Autodesk Fusion 360 part; units mm, degrees
(part 3 of 10)
sketch "草图3 (7)" plane through (727, 0, 0) normal (1, 0, 0) x (0, 0, -1) in component "R2_Integrated"
  line L0 (-20, 137) -> (-20, 165)
  line L1 (-20, 165) -> (-23, 165)
  line L2 (-23, 165) -> (-24.958, 137)
  line L3 (-24.958, 137) -> (-20, 137)
  dimension "d1011" = 23
  dimension "d1012" = 24.958
  constraint vertical L0
  constraint horizontal L1
  constraint horizontal L3
  measures "d1011" horizontal distance of origin L1.end
  measures "d1012" horizontal distance of origin L2.end
extrude "Drain tongue floor'''" add sketch "草图3 (7)" along normal blind 34 bodies 19 in component "R2_Integrated"
ref_plane "工作平面4" through (727, 0, 0) normal (1, 0, 0) x (0, 1, 0) in component "R2_Integrated"
sketch "草图4 (7)" plane through (727, 0, 0) normal (1, 0, 0) x (0, 0, -1) in component "R2_Integrated"
  line L0 (-20, 137) -> (-20, 165)
  line L1 (-20, 165) -> (-29, 165)
  line L2 (-29, 165) -> (-30.958, 137)
  line L3 (-30.958, 137) -> (-20, 137)
  dimension "d1020" = 29
  dimension "d1021" = 30.958
  constraint vertical L0
  constraint horizontal L1
  constraint horizontal L3
  measures "d1020" horizontal distance of origin L1.end
  measures "d1021" horizontal distance of origin L2.end
extrude "Tongue side rail'''" add sketch "草图4 (7)" along normal blind 3 bodies 19 in component "R2_Integrated"
ref_plane "工作平面5" through (758, 0, 0) normal (1, 0, 0) x (0, 1, 0) in component "R2_Integrated"
sketch "草图5 (7)" plane through (758, 0, 0) normal (1, 0, 0) x (0, 0, -1) in component "R2_Integrated"
  line L0 (-20, 137) -> (-20, 165)
  line L1 (-20, 165) -> (-29, 165)
  line L2 (-29, 165) -> (-30.958, 137)
  line L3 (-30.958, 137) -> (-20, 137)
  dimension "d1029" = 29
  dimension "d1030" = 30.958
  constraint vertical L0
  constraint horizontal L1
  constraint horizontal L3
  measures "d1029" horizontal distance of origin L1.end
  measures "d1030" horizontal distance of origin L2.end
extrude "Tongue side rail (1)'''" add sketch "草图5 (7)" along normal blind 3 bodies 19 in component "R2_Integrated"
ref_plane "工作平面6" through (730, 0, 0) normal (1, 0, 0) x (0, 1, 0) in component "R2_Integrated"
sketch "草图6 (7)" plane through (730, 0, 0) normal (1, 0, 0) x (0, 0, -1) in component "R2_Integrated"
  line L0 (-24.958, 137) -> (-23, 165)
  line L1 (-23, 165) -> (-41, 165)
  line L2 (-41, 165) -> (-41, 137)
  line L3 (-41, 137) -> (-24.958, 137)
  dimension "d1035" = 24.958
  dimension "d1037" = 23
  dimension "d1039" = 41
  constraint horizontal L1
  constraint vertical L2
  constraint horizontal L3
  measures "d1035" horizontal distance of origin L0.start
  measures "d1037" horizontal distance of origin L0.end
  measures "d1039" horizontal distance of origin L1.end
extrude "Open drain mouth'''" cut sketch "草图6 (7)" along normal blind 28 bodies 19 in component "R2_Integrated"
ref_plane "工作平面7" through (0, 0, 20) normal (0, 0, 1) x (1, 0, 0) in component "R2_Integrated"
sketch "草图7 (7)" plane through (0, 0, 20) normal (0, 0, 1) x (1, 0, 0) in component "R2_Integrated"
  line L0 (729, 53) -> (741, 53)
  line L1 (741, 53) -> (741, 65)
  line L2 (741, 65) -> (729, 65)
  line L3 (729, 65) -> (729, 53)
  dimension "d1044" = 729
  dimension "d1046" = 12
  dimension "d1047" = 12
  constraint horizontal L0
  constraint vertical L1
  constraint horizontal L2
  constraint vertical L3
  measures "d1044" horizontal distance of origin L0.start
  measures "d1046" horizontal distance of L0.start L0.end
  measures "d1047" vertical distance of L0.end L1.end
extrude "Grate seat 00'''" add sketch "草图7 (7)" along normal blind 16 bodies 19 in component "R2_Integrated"
ref_plane "工作平面8" through (0, 0, 20) normal (0, 0, 1) x (1, 0, 0) in component "R2_Integrated"
sketch "草图8 (7)" plane through (0, 0, 20) normal (0, 0, 1) x (1, 0, 0) in component "R2_Integrated"
  line L0 (761, 125) -> (773, 125)
  line L1 (773, 125) -> (773, 137)
  line L2 (773, 137) -> (761, 137)
  line L3 (761, 137) -> (761, 125)
  dimension "d1052" = 761
  dimension "d1053" = 125
  dimension "d1054" = 12
  dimension "d1055" = 12
  constraint horizontal L0
  constraint vertical L1
  constraint horizontal L2
  constraint vertical L3
  measures "d1052" horizontal distance of origin L0.start
  measures "d1053" vertical distance of origin L0.start
  measures "d1054" horizontal distance of L0.start L0.end
  measures "d1055" vertical distance of L0.end L1.end
extrude "Grate seat 01'''" add sketch "草图8 (7)" along normal blind 16 bodies 19 in component "R2_Integrated"
ref_plane "工作平面9" through (0, 0, 20) normal (0, 0, 1) x (1, 0, 0) in component "R2_Integrated"
sketch "草图9 (7)" plane through (0, 0, 20) normal (0, 0, 1) x (1, 0, 0) in component "R2_Integrated"
  line L0 (845, 53) -> (857, 53)
  line L1 (857, 53) -> (857, 65)
  line L2 (857, 65) -> (845, 65)
  line L3 (845, 65) -> (845, 53)
  dimension "d1060" = 845
  dimension "d1062" = 12
  dimension "d1063" = 12
  constraint horizontal L0
  constraint vertical L1
  constraint horizontal L2
  constraint vertical L3
  measures "d1060" horizontal distance of origin L0.start
  measures "d1062" horizontal distance of L0.start L0.end
  measures "d1063" vertical distance of L0.end L1.end
extrude "Grate seat 10'''" add sketch "草图9 (7)" along normal blind 16 bodies 19 in component "R2_Integrated"
ref_plane "工作平面10" through (0, 0, 20) normal (0, 0, 1) x (1, 0, 0) in component "R2_Integrated"
sketch "草图10 (7)" plane through (0, 0, 20) normal (0, 0, 1) x (1, 0, 0) in component "R2_Integrated"
  line L0 (845, 125) -> (857, 125)
  line L1 (857, 125) -> (857, 137)
  line L2 (857, 137) -> (845, 137)
  line L3 (845, 137) -> (845, 125)
  dimension "d1068" = 845
  dimension "d1069" = 125
  dimension "d1070" = 12
  dimension "d1071" = 12
  constraint horizontal L0
  constraint vertical L1
  constraint horizontal L2
  constraint vertical L3
  measures "d1068" horizontal distance of origin L0.start
  measures "d1069" vertical distance of origin L0.start
  measures "d1070" horizontal distance of L0.start L0.end
  measures "d1071" vertical distance of L0.end L1.end
extrude "Grate seat 11'''" add sketch "草图10 (7)" along normal blind 16 bodies 19 in component "R2_Integrated"
ref_plane "工作平面11" through (727, 0, 0) normal (1, 0, 0) x (0, 1, 0) in component "R2_Integrated"
sketch "草图11 (7)" plane through (727, 0, 0) normal (1, 0, 0) x (0, 0, -1) in component "R2_Integrated"
  line L0 (-19.8, 163) -> (-19.8, 164)
  line L1 (-19.8, 164) -> (-20.6, 164)
  line L2 (-20.6, 164) -> (-20.6, 163)
  line L3 (-20.6, 163) -> (-19.8, 163)
  dimension "d1076" = 19.8
  dimension "d1077" = 163
  dimension "d1078" = 164
  dimension "d1079" = 20.6
  constraint vertical L0
  constraint horizontal L1
  constraint vertical L2
  constraint horizontal L3
  measures "d1076" horizontal distance of origin L0.start
  measures "d1077" vertical distance of origin L0.start
  measures "d1078" vertical distance of origin L0.end
  measures "d1079" horizontal distance of origin L1.end
extrude "Drip break underside groove'''" cut sketch "草图11 (7)" along normal blind 34 bodies 19 in component "R2_Integrated"
ref_plane "工作平面12" through (0, 0, 20) normal (0, 0, 1) x (1, 0, 0) in component "R2_Integrated"
sketch "草图12 (7)" plane through (0, 0, 20) normal (0, 0, 1) x (1, 0, 0) in component "R2_Integrated"
  line L0 (732.75, 56.75) -> (741.25, 56.75)
  line L1 (741.25, 56.75) -> (741.25, 65.25)
  line L2 (741.25, 65.25) -> (732.75, 65.25)
  line L3 (732.75, 65.25) -> (732.75, 56.75)
  dimension "d1084" = 732.75
  dimension "d1085" = 56.75
  dimension "d1086" = 8.5
  dimension "d1087" = 8.5
  constraint horizontal L0
  constraint vertical L1
  constraint horizontal L2
  constraint vertical L3
  measures "d1084" horizontal distance of origin L0.start
  measures "d1085" vertical distance of origin L0.start
  measures "d1086" horizontal distance of L0.start L0.end
  measures "d1087" vertical distance of L0.end L1.end
extrude "Foot socket 00'''" cut sketch "草图12 (7)" along normal blind 1.8 bodies 19 in component "R2_Integrated"
ref_plane "工作平面13" through (0, 0, 20) normal (0, 0, 1) x (1, 0, 0) in component "R2_Integrated"
sketch "草图13 (7)" plane through (0, 0, 20) normal (0, 0, 1) x (1, 0, 0) in component "R2_Integrated"
  line L0 (732.75, 118.75) -> (741.25, 118.75)
  line L1 (741.25, 118.75) -> (741.25, 127.25)
  line L2 (741.25, 127.25) -> (732.75, 127.25)
  line L3 (732.75, 127.25) -> (732.75, 118.75)
  dimension "d1092" = 732.75
  dimension "d1093" = 118.75
  dimension "d1094" = 8.5
  dimension "d1095" = 8.5
  constraint horizontal L0
  constraint vertical L1
  constraint horizontal L2
  constraint vertical L3
  measures "d1092" horizontal distance of origin L0.start
  measures "d1093" vertical distance of origin L0.start
  measures "d1094" horizontal distance of L0.start L0.end
  measures "d1095" vertical distance of L0.end L1.end
extrude "Foot socket 01'''" cut sketch "草图13 (7)" along normal blind 1.8 bodies 19 in component "R2_Integrated"
ref_plane "工作平面14" through (0, 0, 20) normal (0, 0, 1) x (1, 0, 0) in component "R2_Integrated"
sketch "草图14 (6)" plane through (0, 0, 20) normal (0, 0, 1) x (1, 0, 0) in component "R2_Integrated"
  line L0 (844.75, 56.75) -> (853.25, 56.75)
  line L1 (853.25, 56.75) -> (853.25, 65.25)
  line L2 (853.25, 65.25) -> (844.75, 65.25)
  line L3 (844.75, 65.25) -> (844.75, 56.75)
  dimension "d1100" = 844.75
  dimension "d1101" = 56.75
  dimension "d1102" = 8.5
  dimension "d1103" = 8.5
  constraint horizontal L0
  constraint vertical L1
  constraint horizontal L2
  constraint vertical L3
  measures "d1100" horizontal distance of origin L0.start
  measures "d1101" vertical distance of origin L0.start
  measures "d1102" horizontal distance of L0.start L0.end
  measures "d1103" vertical distance of L0.end L1.end
extrude "Foot socket 10'''" cut sketch "草图14 (6)" along normal blind 1.8 bodies 19 in component "R2_Integrated"
ref_plane "工作平面15" through (0, 0, 20) normal (0, 0, 1) x (1, 0, 0) in component "R2_Integrated"
sketch "草图15 (6)" plane through (0, 0, 20) normal (0, 0, 1) x (1, 0, 0) in component "R2_Integrated"
  line L0 (844.75, 118.75) -> (853.25, 118.75)
  line L1 (853.25, 118.75) -> (853.25, 127.25)
  line L2 (853.25, 127.25) -> (844.75, 127.25)
  line L3 (844.75, 127.25) -> (844.75, 118.75)
  dimension "d1108" = 844.75
  dimension "d1109" = 118.75
  dimension "d1110" = 8.5
  dimension "d1111" = 8.5
  constraint horizontal L0
  constraint vertical L1
  constraint horizontal L2
  constraint vertical L3
  measures "d1108" horizontal distance of origin L0.start
  measures "d1109" vertical distance of origin L0.start
  measures "d1110" horizontal distance of L0.start L0.end
  measures "d1111" vertical distance of L0.end L1.end
extrude "Foot socket 11'''" cut sketch "草图15 (6)" along normal blind 1.8 bodies 19 in component "R2_Integrated"
ref_plane "工作平面1" through (0, 0, 36) normal (0, 0, 1) x (1, 0, 0) in component "R2_RemovableGrate"
sketch "草图1 (20)" plane through (0, 0, 36) normal (0, 0, 1) x (1, 0, 0) in component "R2_RemovableGrate"
  line L0 (729.3, 53.3) -> (856.7, 53.3)
  line L1 (856.7, 53.3) -> (856.7, 136.7)
  line L2 (856.7, 136.7) -> (729.3, 136.7)
  line L3 (729.3, 136.7) -> (729.3, 53.3)
  dimension "d1116" = 729.3
  dimension "d1118" = 127.4
  dimension "d1119" = 83.4
  constraint horizontal L0
  constraint vertical L1
  constraint horizontal L2
  constraint vertical L3
  measures "d1116" horizontal distance of origin L0.start
  measures "d1118" horizontal distance of L0.start L0.end
  measures "d1119" vertical distance of L0.end L1.end
extrude "Horizontal removable deck'''" add sketch "草图1 (20)" along normal blind 4 separate body makes body 20 in component "R2_RemovableGrate"
ref_plane "工作平面2" through (0, 0, 36) normal (0, 0, 1) x (1, 0, 0) in component "R2_RemovableGrate"
sketch "草图2 (20)" plane through (0, 0, 36) normal (0, 0, 1) x (1, 0, 0) in component "R2_RemovableGrate"
  line L0 (741, 60.3) -> (745, 60.3)
  line L1 (745, 60.3) -> (745, 129.7)
  line L2 (745, 129.7) -> (741, 129.7)
  line L3 (741, 129.7) -> (741, 60.3)
  dimension "d1124" = 741
  dimension "d1126" = 4
  dimension "d1127" = 69.4
  constraint horizontal L0
  constraint vertical L1
  constraint horizontal L2
  constraint vertical L3
  measures "d1124" horizontal distance of origin L0.start
  measures "d1126" horizontal distance of L0.start L0.end
  measures "d1127" vertical distance of L0.end L1.end
extrude "Drain slot 1'''" cut sketch "草图2 (20)" along normal blind 4 bodies 20 in component "R2_RemovableGrate"
ref_plane "工作平面3" through (0, 0, 36) normal (0, 0, 1) x (1, 0, 0) in component "R2_RemovableGrate"
sketch "草图3 (8)" plane through (0, 0, 36) normal (0, 0, 1) x (1, 0, 0) in component "R2_RemovableGrate"
  line L0 (751, 60.3) -> (755, 60.3)
  line L1 (755, 60.3) -> (755, 129.7)
  line L2 (755, 129.7) -> (751, 129.7)
  line L3 (751, 129.7) -> (751, 60.3)
  dimension "d1132" = 751
  dimension "d1134" = 4
  dimension "d1135" = 69.4
  constraint horizontal L0
  constraint vertical L1
  constraint horizontal L2
  constraint vertical L3
  measures "d1132" horizontal distance of origin L0.start
  measures "d1134" horizontal distance of L0.start L0.end
  measures "d1135" vertical distance of L0.end L1.end
extrude "Drain slot 2'''" cut sketch "草图3 (8)" along normal blind 4 bodies 20 in component "R2_RemovableGrate"
ref_plane "工作平面4" through (0, 0, 36) normal (0, 0, 1) x (1, 0, 0) in component "R2_RemovableGrate"
sketch "草图4 (8)" plane through (0, 0, 36) normal (0, 0, 1) x (1, 0, 0) in component "R2_RemovableGrate"
  line L0 (761, 60.3) -> (765, 60.3)
  line L1 (765, 60.3) -> (765, 129.7)
  line L2 (765, 129.7) -> (761, 129.7)
  line L3 (761, 129.7) -> (761, 60.3)
  dimension "d1140" = 761
  dimension "d1142" = 4
  dimension "d1143" = 69.4
  constraint horizontal L0
  constraint vertical L1
  constraint horizontal L2
  constraint vertical L3
  measures "d1140" horizontal distance of origin L0.start
  measures "d1142" horizontal distance of L0.start L0.end
  measures "d1143" vertical distance of L0.end L1.end
extrude "Drain slot 3'''" cut sketch "草图4 (8)" along normal blind 4 bodies 20 in component "R2_RemovableGrate"
ref_plane "工作平面5" through (0, 0, 36) normal (0, 0, 1) x (1, 0, 0) in component "R2_RemovableGrate"
sketch "草图5 (8)" plane through (0, 0, 36) normal (0, 0, 1) x (1, 0, 0) in component "R2_RemovableGrate"
  line L0 (771, 60.3) -> (775, 60.3)
  line L1 (775, 60.3) -> (775, 129.7)
  line L2 (775, 129.7) -> (771, 129.7)
  line L3 (771, 129.7) -> (771, 60.3)
  dimension "d1148" = 771
  dimension "d1150" = 4
  dimension "d1151" = 69.4
  constraint horizontal L0
  constraint vertical L1
  constraint horizontal L2
  constraint vertical L3
  measures "d1148" horizontal distance of origin L0.start
  measures "d1150" horizontal distance of L0.start L0.end
  measures "d1151" vertical distance of L0.end L1.end
extrude "Drain slot 4'''" cut sketch "草图5 (8)" along normal blind 4 bodies 20 in component "R2_RemovableGrate"
ref_plane "工作平面6" through (0, 0, 36) normal (0, 0, 1) x (1, 0, 0) in component "R2_RemovableGrate"
sketch "草图6 (8)" plane through (0, 0, 36) normal (0, 0, 1) x (1, 0, 0) in component "R2_RemovableGrate"
  line L0 (781, 60.3) -> (785, 60.3)
  line L1 (785, 60.3) -> (785, 129.7)
  line L2 (785, 129.7) -> (781, 129.7)
  line L3 (781, 129.7) -> (781, 60.3)
  dimension "d1156" = 781
  dimension "d1158" = 4
  dimension "d1159" = 69.4
  constraint horizontal L0
  constraint vertical L1
  constraint horizontal L2
  constraint vertical L3
  measures "d1156" horizontal distance of origin L0.start
  measures "d1158" horizontal distance of L0.start L0.end
  measures "d1159" vertical distance of L0.end L1.end
extrude "Drain slot 5'''" cut sketch "草图6 (8)" along normal blind 4 bodies 20 in component "R2_RemovableGrate"
ref_plane "工作平面7" through (0, 0, 36) normal (0, 0, 1) x (1, 0, 0) in component "R2_RemovableGrate"
sketch "草图7 (8)" plane through (0, 0, 36) normal (0, 0, 1) x (1, 0, 0) in component "R2_RemovableGrate"
  line L0 (791, 60.3) -> (795, 60.3)
  line L1 (795, 60.3) -> (795, 129.7)
  line L2 (795, 129.7) -> (791, 129.7)
  line L3 (791, 129.7) -> (791, 60.3)
  dimension "d1164" = 791
  dimension "d1166" = 4
  dimension "d1167" = 69.4
  constraint horizontal L0
  constraint vertical L1
  constraint horizontal L2
  constraint vertical L3
  measures "d1164" horizontal distance of origin L0.start
  measures "d1166" horizontal distance of L0.start L0.end
  measures "d1167" vertical distance of L0.end L1.end
extrude "Drain slot 6'''" cut sketch "草图7 (8)" along normal blind 4 bodies 20 in component "R2_RemovableGrate"
ref_plane "工作平面8" through (0, 0, 36) normal (0, 0, 1) x (1, 0, 0) in component "R2_RemovableGrate"
sketch "草图8 (8)" plane through (0, 0, 36) normal (0, 0, 1) x (1, 0, 0) in component "R2_RemovableGrate"
  line L0 (801, 60.3) -> (805, 60.3)
  line L1 (805, 60.3) -> (805, 129.7)
  line L2 (805, 129.7) -> (801, 129.7)
  line L3 (801, 129.7) -> (801, 60.3)
  dimension "d1172" = 801
  dimension "d1174" = 4
  dimension "d1175" = 69.4
  constraint horizontal L0
  constraint vertical L1
  constraint horizontal L2
  constraint vertical L3
  measures "d1172" horizontal distance of origin L0.start
  measures "d1174" horizontal distance of L0.start L0.end
  measures "d1175" vertical distance of L0.end L1.end
extrude "Drain slot 7'''" cut sketch "草图8 (8)" along normal blind 4 bodies 20 in component "R2_RemovableGrate"
ref_plane "工作平面9" through (0, 0, 36) normal (0, 0, 1) x (1, 0, 0) in component "R2_RemovableGrate"
sketch "草图9 (8)" plane through (0, 0, 36) normal (0, 0, 1) x (1, 0, 0) in component "R2_RemovableGrate"
  line L0 (811, 60.3) -> (815, 60.3)
  line L1 (815, 60.3) -> (815, 129.7)
  line L2 (815, 129.7) -> (811, 129.7)
  line L3 (811, 129.7) -> (811, 60.3)
  dimension "d1180" = 811
  dimension "d1182" = 4
  dimension "d1183" = 69.4
  constraint horizontal L0
  constraint vertical L1
  constraint horizontal L2
  constraint vertical L3
  measures "d1180" horizontal distance of origin L0.start
  measures "d1182" horizontal distance of L0.start L0.end
  measures "d1183" vertical distance of L0.end L1.end
extrude "Drain slot 8'''" cut sketch "草图9 (8)" along normal blind 4 bodies 20 in component "R2_RemovableGrate"
ref_plane "工作平面10" through (0, 0, 36) normal (0, 0, 1) x (1, 0, 0) in component "R2_RemovableGrate"
sketch "草图10 (8)" plane through (0, 0, 36) normal (0, 0, 1) x (1, 0, 0) in component "R2_RemovableGrate"
  line L0 (821, 60.3) -> (825, 60.3)
  line L1 (825, 60.3) -> (825, 129.7)
  line L2 (825, 129.7) -> (821, 129.7)
  line L3 (821, 129.7) -> (821, 60.3)
  dimension "d1188" = 821
  dimension "d1190" = 4
  dimension "d1191" = 69.4
  constraint horizontal L0
  constraint vertical L1
  constraint horizontal L2
  constraint vertical L3
  measures "d1188" horizontal distance of origin L0.start
  measures "d1190" horizontal distance of L0.start L0.end
  measures "d1191" vertical distance of L0.end L1.end
extrude "Drain slot 9'''" cut sketch "草图10 (8)" along normal blind 4 bodies 20 in component "R2_RemovableGrate"
ref_plane "工作平面11" through (0, 0, 36) normal (0, 0, 1) x (1, 0, 0) in component "R2_RemovableGrate"
sketch "草图11 (8)" plane through (0, 0, 36) normal (0, 0, 1) x (1, 0, 0) in component "R2_RemovableGrate"
  line L0 (831, 60.3) -> (835, 60.3)
  line L1 (835, 60.3) -> (835, 129.7)
  line L2 (835, 129.7) -> (831, 129.7)
  line L3 (831, 129.7) -> (831, 60.3)
  dimension "d1196" = 831
  dimension "d1198" = 4
  dimension "d1199" = 69.4
  constraint horizontal L0
  constraint vertical L1
  constraint horizontal L2
  constraint vertical L3
  measures "d1196" horizontal distance of origin L0.start
  measures "d1198" horizontal distance of L0.start L0.end
  measures "d1199" vertical distance of L0.end L1.end
extrude "Drain slot 10'''" cut sketch "草图11 (8)" along normal blind 4 bodies 20 in component "R2_RemovableGrate"
ref_plane "工作平面12" through (0, 0, 36) normal (0, 0, 1) x (1, 0, 0) in component "R2_RemovableGrate"
sketch "草图12 (8)" plane through (0, 0, 36) normal (0, 0, 1) x (1, 0, 0) in component "R2_RemovableGrate"
  line L0 (841, 60.3) -> (845, 60.3)
  line L1 (845, 60.3) -> (845, 129.7)
  line L2 (845, 129.7) -> (841, 129.7)
  line L3 (841, 129.7) -> (841, 60.3)
  dimension "d1204" = 841
  dimension "d1206" = 4
  dimension "d1207" = 69.4
  constraint horizontal L0
  constraint vertical L1
  constraint horizontal L2
  constraint vertical L3
  measures "d1204" horizontal distance of origin L0.start
  measures "d1206" horizontal distance of L0.start L0.end
  measures "d1207" vertical distance of L0.end L1.end
extrude "Drain slot 11'''" cut sketch "草图12 (8)" along normal blind 4 bodies 20 in component "R2_RemovableGrate"
ref_plane "工作平面13" through (0, 0, 36) normal (0, 0, 1) x (1, 0, 0) in component "R2_RemovableGrate"
sketch "草图13 (8)" plane through (0, 0, 36) normal (0, 0, 1) x (1, 0, 0) in component "R2_RemovableGrate"
  line L0 (785, 132.7) -> (801, 132.7)
  line L1 (801, 132.7) -> (801, 137.7)
  line L2 (801, 137.7) -> (785, 137.7)
  line L3 (785, 137.7) -> (785, 132.7)
  dimension "d1212" = 785
  dimension "d1213" = 132.7
  dimension "d1214" = 16
  dimension "d1215" = 5
  constraint horizontal L0
  constraint vertical L1
  constraint horizontal L2
  constraint vertical L3
  measures "d1212" horizontal distance of origin L0.start
  measures "d1213" vertical distance of origin L0.start
  measures "d1214" horizontal distance of L0.start L0.end
  measures "d1215" vertical distance of L0.end L1.end
extrude "Finger lift notch'''" cut sketch "草图13 (8)" along normal blind 4 bodies 20 in component "R2_RemovableGrate"
ref_plane "工作平面1" through (0, 0, 0) normal (0, 0, 1) x (1, 0, 0) in component "R2_Foot_00"
sketch "草图1 (21)" plane through (0, 0, 0) normal (0, 0, 1) x (1, 0, 0) in component "R2_Foot_00"
  line L0 (729, 53) -> (745, 53)
  line L1 (745, 53) -> (745, 69)
  line L2 (745, 69) -> (729, 69)
  line L3 (729, 69) -> (729, 53)
  dimension "d1220" = 729
  dimension "d1221" = 53
  dimension "d1222" = 16
  dimension "d1223" = 16
  constraint horizontal L0
  constraint vertical L1
  constraint horizontal L2
  constraint vertical L3
  measures "d1220" horizontal distance of origin L0.start
  measures "d1221" vertical distance of origin L0.start
  measures "d1222" horizontal distance of L0.start L0.end
  measures "d1223" vertical distance of L0.end L1.end
extrude "Foot base''''''''''''" add sketch "草图1 (21)" along normal blind 20 separate body makes body 21 in component "R2_Foot_00"
ref_plane "工作平面2" through (0, 0, 20) normal (0, 0, 1) x (1, 0, 0) in component "R2_Foot_00"
sketch "草图2 (21)" plane through (0, 0, 20) normal (0, 0, 1) x (1, 0, 0) in component "R2_Foot_00"
  line L0 (733, 57) -> (741, 57)
  line L1 (741, 57) -> (741, 65)
  line L2 (741, 65) -> (733, 65)
  line L3 (733, 65) -> (733, 57)
  dimension "d1228" = 733
  dimension "d1229" = 57
  dimension "d1230" = 8
  dimension "d1231" = 8
  constraint horizontal L0
  constraint vertical L1
  constraint horizontal L2
  constraint vertical L3
  measures "d1228" horizontal distance of origin L0.start
  measures "d1229" vertical distance of origin L0.start
  measures "d1230" horizontal distance of L0.start L0.end
  measures "d1231" vertical distance of L0.end L1.end
extrude "Locating peg''''''''''''" add sketch "草图2 (21)" along normal blind 1.5 bodies 21 in component "R2_Foot_00"
ref_plane "工作平面1" through (0, 0, 0) normal (0, 0, 1) x (1, 0, 0) in component "R2_Foot_01"
sketch "草图1 (22)" plane through (0, 0, 0) normal (0, 0, 1) x (1, 0, 0) in component "R2_Foot_01"
  line L0 (729, 115) -> (745, 115)
  line L1 (745, 115) -> (745, 131)
  line L2 (745, 131) -> (729, 131)
  line L3 (729, 131) -> (729, 115)
  dimension "d1236" = 729
  dimension "d1237" = 115
  dimension "d1238" = 16
  dimension "d1239" = 16
  constraint horizontal L0
  constraint vertical L1
  constraint horizontal L2
  constraint vertical L3
  measures "d1236" horizontal distance of origin L0.start
  measures "d1237" vertical distance of origin L0.start
  measures "d1238" horizontal distance of L0.start L0.end
  measures "d1239" vertical distance of L0.end L1.end
extrude "Foot base'''''''''''''" add sketch "草图1 (22)" along normal blind 20 separate body makes body 22 in component "R2_Foot_01"
ref_plane "工作平面2" through (0, 0, 20) normal (0, 0, 1) x (1, 0, 0) in component "R2_Foot_01"
sketch "草图2 (22)" plane through (0, 0, 20) normal (0, 0, 1) x (1, 0, 0) in component "R2_Foot_01"
  line L0 (733, 119) -> (741, 119)
  line L1 (741, 119) -> (741, 127)
  line L2 (741, 127) -> (733, 127)
  line L3 (733, 127) -> (733, 119)
  dimension "d1244" = 733
  dimension "d1245" = 119
  dimension "d1246" = 8
  dimension "d1247" = 8
  constraint horizontal L0
  constraint vertical L1
  constraint horizontal L2
  constraint vertical L3
  measures "d1244" horizontal distance of origin L0.start
  measures "d1245" vertical distance of origin L0.start
  measures "d1246" horizontal distance of L0.start L0.end
  measures "d1247" vertical distance of L0.end L1.end
extrude "Locating peg'''''''''''''" add sketch "草图2 (22)" along normal blind 1.5 bodies 22 in component "R2_Foot_01"
ref_plane "工作平面1" through (0, 0, 0) normal (0, 0, 1) x (1, 0, 0) in component "R2_Foot_10"
sketch "草图1 (23)" plane through (0, 0, 0) normal (0, 0, 1) x (1, 0, 0) in component "R2_Foot_10"
  line L0 (841, 53) -> (857, 53)
  line L1 (857, 53) -> (857, 69)
  line L2 (857, 69) -> (841, 69)
  line L3 (841, 69) -> (841, 53)
  dimension "d1252" = 841
  dimension "d1253" = 53
  dimension "d1254" = 16
  dimension "d1255" = 16
  constraint horizontal L0
  constraint vertical L1
  constraint horizontal L2
  constraint vertical L3
  measures "d1252" horizontal distance of origin L0.start
  measures "d1253" vertical distance of origin L0.start
  measures "d1254" horizontal distance of L0.start L0.end
  measures "d1255" vertical distance of L0.end L1.end
extrude "Foot base''''''''''''''" add sketch "草图1 (23)" along normal blind 20 separate body makes body 23 in component "R2_Foot_10"
ref_plane "工作平面2" through (0, 0, 20) normal (0, 0, 1) x (1, 0, 0) in component "R2_Foot_10"
sketch "草图2 (23)" plane through (0, 0, 20) normal (0, 0, 1) x (1, 0, 0) in component "R2_Foot_10"
  line L0 (845, 57) -> (853, 57)
  line L1 (853, 57) -> (853, 65)
  line L2 (853, 65) -> (845, 65)
  line L3 (845, 65) -> (845, 57)
  dimension "d1260" = 845
  dimension "d1261" = 57
  dimension "d1262" = 8
  dimension "d1263" = 8
  constraint horizontal L0
  constraint vertical L1
  constraint horizontal L2
  constraint vertical L3
  measures "d1260" horizontal distance of origin L0.start
  measures "d1261" vertical distance of origin L0.start
  measures "d1262" horizontal distance of L0.start L0.end
  measures "d1263" vertical distance of L0.end L1.end
extrude "Locating peg''''''''''''''" add sketch "草图2 (23)" along normal blind 1.5 bodies 23 in component "R2_Foot_10"
ref_plane "工作平面1" through (0, 0, 0) normal (0, 0, 1) x (1, 0, 0) in component "R2_Foot_11"
sketch "草图1 (24)" plane through (0, 0, 0) normal (0, 0, 1) x (1, 0, 0) in component "R2_Foot_11"
  line L0 (841, 115) -> (857, 115)
  line L1 (857, 115) -> (857, 131)
  line L2 (857, 131) -> (841, 131)
  line L3 (841, 131) -> (841, 115)
  dimension "d1268" = 841
  dimension "d1269" = 115
  dimension "d1270" = 16
  dimension "d1271" = 16
  constraint horizontal L0
  constraint vertical L1
  constraint horizontal L2
  constraint vertical L3
  measures "d1268" horizontal distance of origin L0.start
  measures "d1269" vertical distance of origin L0.start
  measures "d1270" horizontal distance of L0.start L0.end
  measures "d1271" vertical distance of L0.end L1.end
extrude "Foot base'''''''''''''''" add sketch "草图1 (24)" along normal blind 20 separate body makes body 24 in component "R2_Foot_11"
ref_plane "工作平面2" through (0, 0, 20) normal (0, 0, 1) x (1, 0, 0) in component "R2_Foot_11"
sketch "草图2 (24)" plane through (0, 0, 20) normal (0, 0, 1) x (1, 0, 0) in component "R2_Foot_11"
  line L0 (845, 119) -> (853, 119)
  line L1 (853, 119) -> (853, 127)
  line L2 (853, 127) -> (845, 127)
  line L3 (845, 127) -> (845, 119)
  dimension "d1276" = 845
  dimension "d1277" = 119
  dimension "d1278" = 8
  dimension "d1279" = 8
  constraint horizontal L0
  constraint vertical L1
  constraint horizontal L2
  constraint vertical L3
  measures "d1276" horizontal distance of origin L0.start
  measures "d1277" vertical distance of origin L0.start
  measures "d1278" horizontal distance of L0.start L0.end
  measures "d1279" vertical distance of L0.end L1.end
extrude "Locating peg'''''''''''''''" add sketch "草图2 (24)" along normal blind 1.5 bodies 24 in component "R2_Foot_11"
ref_plane "工作平面1" through (0, 0, 20) normal (0, 0, 1) x (1, 0, 0) in component "LS_Integrated"
sketch "草图1 (25)" plane through (0, 0, 20) normal (0, 0, 1) x (1, 0, 0) in component "LS_Integrated"
  line L0 (50, 142) -> (170, 142)
  line L1 (170, 142) -> (170, 322)
  line L2 (170, 322) -> (50, 322)
  line L3 (50, 322) -> (50, 142)
  dimension "d1284" = 50
  dimension "d1285" = 142
  dimension "d1286" = 120
  dimension "d1287" = 180
  constraint horizontal L0
  constraint vertical L1
  constraint horizontal L2
  constraint vertical L3
  measures "d1284" horizontal distance of origin L0.start
  measures "d1285" vertical distance of origin L0.start
  measures "d1286" horizontal distance of L0.start L0.end
  measures "d1287" vertical distance of L0.end L1.end
extrude "Pan blank''''" add sketch "草图1 (25)" along normal blind 20 separate body makes body 25 in component "LS_Integrated"
fillet "Outside corner rounds''''" radius 3 4 edges at (50, 322, 30) (170, 322, 30) (170, 142, 30) (50, 142, 30) on bodies 25 in component "LS_Integrated"
ref_plane "工作平面2" through (0, 319, 0) normal (0, 1, 0) x (0, 0, 1) in component "LS_Integrated"
sketch "草图2 (25)" plane through (0, 319, 0) normal (0, 1, 0) x (1, 0, 0) in component "LS_Integrated"
  line L0 (53, -32.9296) -> (167, -24.958)
  line L1 (167, -24.958) -> (167, -41)
  line L2 (167, -41) -> (53, -41)
  line L3 (53, -41) -> (53, -32.9296)
  dimension "d1295" = 32.9296
  dimension "d1297" = 24.958
  dimension "d1298" = 41
  constraint vertical L1
  constraint horizontal L2
  constraint vertical L3
  measures "d1295" vertical distance of origin L0.start
  measures "d1297" vertical distance of origin L0.end
  measures "d1298" vertical distance of origin L1.end
extrude "Sloped catch cavity''''" cut sketch "草图2 (25)" against normal blind 174 bodies 25 in component "LS_Integrated"
ref_plane "工作平面3" through (0, 249, 0) normal (0, 1, 0) x (0, 0, 1) in component "LS_Integrated"
sketch "草图3 (9)" plane through (0, 249, 0) normal (0, 1, 0) x (1, 0, 0) in component "LS_Integrated"
  line L0 (167, -20) -> (195, -20)
  line L1 (195, -20) -> (195, -23)
  line L2 (195, -23) -> (167, -24.958)
  line L3 (167, -24.958) -> (167, -20)
  dimension "d1306" = 23
  dimension "d1307" = 24.958
  constraint horizontal L0
  constraint vertical L1
  constraint vertical L3
  measures "d1306" vertical distance of origin L1.end
  measures "d1307" vertical distance of origin L2.end
extrude "Drain tongue floor''''" add sketch "草图3 (9)" against normal blind 34 bodies 25 in component "LS_Integrated"
ref_plane "工作平面4" through (0, 249, 0) normal (0, 1, 0) x (0, 0, 1) in component "LS_Integrated"
sketch "草图4 (9)" plane through (0, 249, 0) normal (0, 1, 0) x (1, 0, 0) in component "LS_Integrated"
  line L0 (167, -20) -> (195, -20)
  line L1 (195, -20) -> (195, -29)
  line L2 (195, -29) -> (167, -30.958)
  line L3 (167, -30.958) -> (167, -20)
  dimension "d1315" = 29
  dimension "d1316" = 30.958
  constraint horizontal L0
  constraint vertical L1
  constraint vertical L3
  measures "d1315" vertical distance of origin L1.end
  measures "d1316" vertical distance of origin L2.end
extrude "Tongue side rail''''" add sketch "草图4 (9)" against normal blind 3 bodies 25 in component "LS_Integrated"
ref_plane "工作平面5" through (0, 218, 0) normal (0, 1, 0) x (0, 0, 1) in component "LS_Integrated"
sketch "草图5 (9)" plane through (0, 218, 0) normal (0, 1, 0) x (1, 0, 0) in component "LS_Integrated"
  line L0 (167, -20) -> (195, -20)
  line L1 (195, -20) -> (195, -29)
  line L2 (195, -29) -> (167, -30.958)
  line L3 (167, -30.958) -> (167, -20)
  dimension "d1324" = 29
  dimension "d1325" = 30.958
  constraint horizontal L0
  constraint vertical L1
  constraint vertical L3
  measures "d1324" vertical distance of origin L1.end
  measures "d1325" vertical distance of origin L2.end
extrude "Tongue side rail (1)''''" add sketch "草图5 (9)" against normal blind 3 bodies 25 in component "LS_Integrated"
ref_plane "工作平面6" through (0, 246, 0) normal (0, 1, 0) x (0, 0, 1) in component "LS_Integrated"
sketch "草图6 (9)" plane through (0, 246, 0) normal (0, 1, 0) x (1, 0, 0) in component "LS_Integrated"
  line L0 (167, -24.958) -> (195, -23)
  line L1 (195, -23) -> (195, -41)
  line L2 (195, -41) -> (167, -41)
  line L3 (167, -41) -> (167, -24.958)
  dimension "d1331" = 24.958
  dimension "d1333" = 23
  dimension "d1334" = 41
  constraint vertical L1
  constraint horizontal L2
  constraint vertical L3
  measures "d1331" vertical distance of origin L0.start
  measures "d1333" vertical distance of origin L0.end
  measures "d1334" vertical distance of origin L1.end
extrude "Open drain mouth''''" cut sketch "草图6 (9)" against normal blind 28 bodies 25 in component "LS_Integrated"
ref_plane "工作平面7" through (0, 0, 20) normal (0, 0, 1) x (1, 0, 0) in component "LS_Integrated"
sketch "草图7 (9)" plane through (0, 0, 20) normal (0, 0, 1) x (1, 0, 0) in component "LS_Integrated"
  line L0 (53, 307) -> (65, 307)
  line L1 (65, 307) -> (65, 319)
  line L2 (65, 319) -> (53, 319)
  line L3 (53, 319) -> (53, 307)
  dimension "d1340" = 307
  dimension "d1341" = 12
  dimension "d1342" = 12
  constraint horizontal L0
  constraint vertical L1
  constraint horizontal L2
  constraint vertical L3
  measures "d1340" vertical distance of origin L0.start
  measures "d1341" horizontal distance of L0.start L0.end
  measures "d1342" vertical distance of L0.end L1.end
extrude "Grate seat 00''''" add sketch "草图7 (9)" along normal blind 16 bodies 25 in component "LS_Integrated"
ref_plane "工作平面8" through (0, 0, 20) normal (0, 0, 1) x (1, 0, 0) in component "LS_Integrated"
sketch "草图8 (9)" plane through (0, 0, 20) normal (0, 0, 1) x (1, 0, 0) in component "LS_Integrated"
  line L0 (155, 307) -> (167, 307)
  line L1 (167, 307) -> (167, 319)
  line L2 (167, 319) -> (155, 319)
  line L3 (155, 319) -> (155, 307)
  dimension "d1347" = 155
  dimension "d1348" = 307
  dimension "d1349" = 12
  dimension "d1350" = 12
  constraint horizontal L0
  constraint vertical L1
  constraint horizontal L2
  constraint vertical L3
  measures "d1347" horizontal distance of origin L0.start
  measures "d1348" vertical distance of origin L0.start
  measures "d1349" horizontal distance of L0.start L0.end
  measures "d1350" vertical distance of L0.end L1.end
extrude "Grate seat 01''''" add sketch "草图8 (9)" along normal blind 16 bodies 25 in component "LS_Integrated"
ref_plane "工作平面9" through (0, 0, 20) normal (0, 0, 1) x (1, 0, 0) in component "LS_Integrated"
sketch "草图9 (9)" plane through (0, 0, 20) normal (0, 0, 1) x (1, 0, 0) in component "LS_Integrated"
  line L0 (53, 145) -> (65, 145)
  line L1 (65, 145) -> (65, 157)
  line L2 (65, 157) -> (53, 157)
  line L3 (53, 157) -> (53, 145)
  dimension "d1356" = 145
  dimension "d1357" = 12
  dimension "d1358" = 12
  constraint horizontal L0
  constraint vertical L1
  constraint horizontal L2
  constraint vertical L3
  measures "d1356" vertical distance of origin L0.start
  measures "d1357" horizontal distance of L0.start L0.end
  measures "d1358" vertical distance of L0.end L1.end
extrude "Grate seat 10''''" add sketch "草图9 (9)" along normal blind 16 bodies 25 in component "LS_Integrated"
ref_plane "工作平面10" through (0, 0, 20) normal (0, 0, 1) x (1, 0, 0) in component "LS_Integrated"
sketch "草图10 (9)" plane through (0, 0, 20) normal (0, 0, 1) x (1, 0, 0) in component "LS_Integrated"
  line L0 (155, 145) -> (167, 145)
  line L1 (167, 145) -> (167, 157)
  line L2 (167, 157) -> (155, 157)
  line L3 (155, 157) -> (155, 145)
  dimension "d1363" = 155
  dimension "d1364" = 145
  dimension "d1365" = 12
  dimension "d1366" = 12
  constraint horizontal L0
  constraint vertical L1
  constraint horizontal L2
  constraint vertical L3
  measures "d1363" horizontal distance of origin L0.start
  measures "d1364" vertical distance of origin L0.start
  measures "d1365" horizontal distance of L0.start L0.end
  measures "d1366" vertical distance of L0.end L1.end
extrude "Grate seat 11''''" add sketch "草图10 (9)" along normal blind 16 bodies 25 in component "LS_Integrated"
ref_plane "工作平面11" through (0, 249, 0) normal (0, 1, 0) x (0, 0, 1) in component "LS_Integrated"
sketch "草图11 (9)" plane through (0, 249, 0) normal (0, 1, 0) x (1, 0, 0) in component "LS_Integrated"
  line L0 (193, -19.8) -> (194, -19.8)
  line L1 (194, -19.8) -> (194, -20.6)
  line L2 (194, -20.6) -> (193, -20.6)
  line L3 (193, -20.6) -> (193, -19.8)
  dimension "d1371" = 193
  dimension "d1372" = 19.8
  dimension "d1373" = 194
  dimension "d1374" = 20.6
  constraint horizontal L0
  constraint vertical L1
  constraint horizontal L2
  constraint vertical L3
  measures "d1371" horizontal distance of origin L0.start
  measures "d1372" vertical distance of origin L0.start
  measures "d1373" horizontal distance of origin L0.end
  measures "d1374" vertical distance of origin L1.end
extrude "Drip break underside groove''''" cut sketch "草图11 (9)" against normal blind 34 bodies 25 in component "LS_Integrated"
ref_plane "工作平面12" through (0, 0, 20) normal (0, 0, 1) x (1, 0, 0) in component "LS_Integrated"
sketch "草图12 (9)" plane through (0, 0, 20) normal (0, 0, 1) x (1, 0, 0) in component "LS_Integrated"
  line L0 (56.75, 306.75) -> (65.25, 306.75)
  line L1 (65.25, 306.75) -> (65.25, 315.25)
  line L2 (65.25, 315.25) -> (56.75, 315.25)
  line L3 (56.75, 315.25) -> (56.75, 306.75)
  dimension "d1379" = 56.75
  dimension "d1380" = 306.75
  dimension "d1381" = 8.5
  dimension "d1382" = 8.5
  constraint horizontal L0
  constraint vertical L1
  constraint horizontal L2
  constraint vertical L3
  measures "d1379" horizontal distance of origin L0.start
  measures "d1380" vertical distance of origin L0.start
  measures "d1381" horizontal distance of L0.start L0.end
  measures "d1382" vertical distance of L0.end L1.end
extrude "Foot socket 00''''" cut sketch "草图12 (9)" along normal blind 1.8 bodies 25 in component "LS_Integrated"
ref_plane "工作平面13" through (0, 0, 20) normal (0, 0, 1) x (1, 0, 0) in component "LS_Integrated"
sketch "草图13 (9)" plane through (0, 0, 20) normal (0, 0, 1) x (1, 0, 0) in component "LS_Integrated"
  line L0 (148.75, 306.75) -> (157.25, 306.75)
  line L1 (157.25, 306.75) -> (157.25, 315.25)
  line L2 (157.25, 315.25) -> (148.75, 315.25)
  line L3 (148.75, 315.25) -> (148.75, 306.75)
  dimension "d1387" = 148.75
  dimension "d1388" = 306.75
  dimension "d1389" = 8.5
  dimension "d1390" = 8.5
  constraint horizontal L0
  constraint vertical L1
  constraint horizontal L2
  constraint vertical L3
  measures "d1387" horizontal distance of origin L0.start
  measures "d1388" vertical distance of origin L0.start
  measures "d1389" horizontal distance of L0.start L0.end
  measures "d1390" vertical distance of L0.end L1.end
extrude "Foot socket 01''''" cut sketch "草图13 (9)" along normal blind 1.8 bodies 25 in component "LS_Integrated"
ref_plane "工作平面14" through (0, 0, 20) normal (0, 0, 1) x (1, 0, 0) in component "LS_Integrated"
sketch "草图14 (7)" plane through (0, 0, 20) normal (0, 0, 1) x (1, 0, 0) in component "LS_Integrated"
  line L0 (56.75, 148.75) -> (65.25, 148.75)
  line L1 (65.25, 148.75) -> (65.25, 157.25)
  line L2 (65.25, 157.25) -> (56.75, 157.25)
  line L3 (56.75, 157.25) -> (56.75, 148.75)
  dimension "d1395" = 56.75
  dimension "d1396" = 148.75
  dimension "d1397" = 8.5
  dimension "d1398" = 8.5
  constraint horizontal L0
  constraint vertical L1
  constraint horizontal L2
  constraint vertical L3
  measures "d1395" horizontal distance of origin L0.start
  measures "d1396" vertical distance of origin L0.start
  measures "d1397" horizontal distance of L0.start L0.end
  measures "d1398" vertical distance of L0.end L1.end
extrude "Foot socket 10''''" cut sketch "草图14 (7)" along normal blind 1.8 bodies 25 in component "LS_Integrated"
ref_plane "工作平面15" through (0, 0, 20) normal (0, 0, 1) x (1, 0, 0) in component "LS_Integrated"
sketch "草图15 (7)" plane through (0, 0, 20) normal (0, 0, 1) x (1, 0, 0) in component "LS_Integrated"
  line L0 (148.75, 148.75) -> (157.25, 148.75)
  line L1 (157.25, 148.75) -> (157.25, 157.25)
  line L2 (157.25, 157.25) -> (148.75, 157.25)
  line L3 (148.75, 157.25) -> (148.75, 148.75)
  dimension "d1403" = 148.75
  dimension "d1404" = 148.75
  dimension "d1405" = 8.5
  dimension "d1406" = 8.5
  constraint horizontal L0
  constraint vertical L1
  constraint horizontal L2
  constraint vertical L3
  measures "d1403" horizontal distance of origin L0.start
  measures "d1404" vertical distance of origin L0.start
  measures "d1405" horizontal distance of L0.start L0.end
  measures "d1406" vertical distance of L0.end L1.end
extrude "Foot socket 11''''" cut sketch "草图15 (7)" along normal blind 1.8 bodies 25 in component "LS_Integrated"
ref_plane "工作平面1" through (0, 0, 36) normal (0, 0, 1) x (1, 0, 0) in component "LS_RemovableGrate"
sketch "草图1 (26)" plane through (0, 0, 36) normal (0, 0, 1) x (1, 0, 0) in component "LS_RemovableGrate"
  line L0 (53.3, 145.3) -> (166.7, 145.3)
  line L1 (166.7, 145.3) -> (166.7, 318.7)
  line L2 (166.7, 318.7) -> (53.3, 318.7)
  line L3 (53.3, 318.7) -> (53.3, 145.3)
  dimension "d1412" = 145.3
  dimension "d1413" = 113.4
  dimension "d1414" = 173.4
  constraint horizontal L0
  constraint vertical L1
  constraint horizontal L2
  constraint vertical L3
  measures "d1412" vertical distance of origin L0.start
  measures "d1413" horizontal distance of L0.start L0.end
  measures "d1414" vertical distance of L0.end L1.end
extrude "Horizontal removable deck''''" add sketch "草图1 (26)" along normal blind 4 separate body makes body 26 in component "LS_RemovableGrate"
ref_plane "工作平面2" through (0, 0, 36) normal (0, 0, 1) x (1, 0, 0) in component "LS_RemovableGrate"
sketch "草图2 (26)" plane through (0, 0, 36) normal (0, 0, 1) x (1, 0, 0) in component "LS_RemovableGrate"
  line L0 (60.3, 300) -> (159.7, 300)
  line L1 (159.7, 300) -> (159.7, 304)
  line L2 (159.7, 304) -> (60.3, 304)
  line L3 (60.3, 304) -> (60.3, 300)
  dimension "d1420" = 300
  dimension "d1421" = 99.4
  dimension "d1422" = 4
  constraint horizontal L0
  constraint vertical L1
  constraint horizontal L2
  constraint vertical L3
  measures "d1420" vertical distance of origin L0.start
  measures "d1421" horizontal distance of L0.start L0.end
  measures "d1422" vertical distance of L0.end L1.end
extrude "Drain slot 1''''" cut sketch "草图2 (26)" along normal blind 4 bodies 26 in component "LS_RemovableGrate"
ref_plane "工作平面3" through (0, 0, 36) normal (0, 0, 1) x (1, 0, 0) in component "LS_RemovableGrate"
sketch "草图3 (10)" plane through (0, 0, 36) normal (0, 0, 1) x (1, 0, 0) in component "LS_RemovableGrate"
  line L0 (60.3, 290) -> (159.7, 290)
  line L1 (159.7, 290) -> (159.7, 294)
  line L2 (159.7, 294) -> (60.3, 294)
  line L3 (60.3, 294) -> (60.3, 290)
  dimension "d1428" = 290
  dimension "d1429" = 99.4
  dimension "d1430" = 4
  constraint horizontal L0
  constraint vertical L1
  constraint horizontal L2
  constraint vertical L3
  measures "d1428" vertical distance of origin L0.start
  measures "d1429" horizontal distance of L0.start L0.end
  measures "d1430" vertical distance of L0.end L1.end
extrude "Drain slot 2''''" cut sketch "草图3 (10)" along normal blind 4 bodies 26 in component "LS_RemovableGrate"
ref_plane "工作平面4" through (0, 0, 36) normal (0, 0, 1) x (1, 0, 0) in component "LS_RemovableGrate"
sketch "草图4 (10)" plane through (0, 0, 36) normal (0, 0, 1) x (1, 0, 0) in component "LS_RemovableGrate"
  line L0 (60.3, 280) -> (159.7, 280)
  line L1 (159.7, 280) -> (159.7, 284)
  line L2 (159.7, 284) -> (60.3, 284)
  line L3 (60.3, 284) -> (60.3, 280)
  dimension "d1436" = 280
  dimension "d1437" = 99.4
  dimension "d1438" = 4
  constraint horizontal L0
  constraint vertical L1
  constraint horizontal L2
  constraint vertical L3
  measures "d1436" vertical distance of origin L0.start
  measures "d1437" horizontal distance of L0.start L0.end
  measures "d1438" vertical distance of L0.end L1.end
extrude "Drain slot 3''''" cut sketch "草图4 (10)" along normal blind 4 bodies 26 in component "LS_RemovableGrate"
ref_plane "工作平面5" through (0, 0, 36) normal (0, 0, 1) x (1, 0, 0) in component "LS_RemovableGrate"
sketch "草图5 (10)" plane through (0, 0, 36) normal (0, 0, 1) x (1, 0, 0) in component "LS_RemovableGrate"
  line L0 (60.3, 270) -> (159.7, 270)
  line L1 (159.7, 270) -> (159.7, 274)
  line L2 (159.7, 274) -> (60.3, 274)
  line L3 (60.3, 274) -> (60.3, 270)
  dimension "d1444" = 270
  dimension "d1445" = 99.4
  dimension "d1446" = 4
  constraint horizontal L0
  constraint vertical L1
  constraint horizontal L2
  constraint vertical L3
  measures "d1444" vertical distance of origin L0.start
  measures "d1445" horizontal distance of L0.start L0.end
  measures "d1446" vertical distance of L0.end L1.end
extrude "Drain slot 4''''" cut sketch "草图5 (10)" along normal blind 4 bodies 26 in component "LS_RemovableGrate"
ref_plane "工作平面6" through (0, 0, 36) normal (0, 0, 1) x (1, 0, 0) in component "LS_RemovableGrate"
sketch "草图6 (10)" plane through (0, 0, 36) normal (0, 0, 1) x (1, 0, 0) in component "LS_RemovableGrate"
  line L0 (60.3, 260) -> (159.7, 260)
  line L1 (159.7, 260) -> (159.7, 264)
  line L2 (159.7, 264) -> (60.3, 264)
  line L3 (60.3, 264) -> (60.3, 260)
  dimension "d1452" = 260
  dimension "d1453" = 99.4
  dimension "d1454" = 4
  constraint horizontal L0
  constraint vertical L1
  constraint horizontal L2
  constraint vertical L3
  measures "d1452" vertical distance of origin L0.start
  measures "d1453" horizontal distance of L0.start L0.end
  measures "d1454" vertical distance of L0.end L1.end
extrude "Drain slot 5''''" cut sketch "草图6 (10)" along normal blind 4 bodies 26 in component "LS_RemovableGrate"
ref_plane "工作平面7" through (0, 0, 36) normal (0, 0, 1) x (1, 0, 0) in component "LS_RemovableGrate"
sketch "草图7 (10)" plane through (0, 0, 36) normal (0, 0, 1) x (1, 0, 0) in component "LS_RemovableGrate"
  line L0 (60.3, 250) -> (159.7, 250)
  line L1 (159.7, 250) -> (159.7, 254)
  line L2 (159.7, 254) -> (60.3, 254)
  line L3 (60.3, 254) -> (60.3, 250)
  dimension "d1460" = 250
  dimension "d1461" = 99.4
  dimension "d1462" = 4
  constraint horizontal L0
  constraint vertical L1
  constraint horizontal L2
  constraint vertical L3
  measures "d1460" vertical distance of origin L0.start
  measures "d1461" horizontal distance of L0.start L0.end
  measures "d1462" vertical distance of L0.end L1.end
extrude "Drain slot 6''''" cut sketch "草图7 (10)" along normal blind 4 bodies 26 in component "LS_RemovableGrate"
ref_plane "工作平面8" through (0, 0, 36) normal (0, 0, 1) x (1, 0, 0) in component "LS_RemovableGrate"
sketch "草图8 (10)" plane through (0, 0, 36) normal (0, 0, 1) x (1, 0, 0) in component "LS_RemovableGrate"
  line L0 (60.3, 240) -> (159.7, 240)
  line L1 (159.7, 240) -> (159.7, 244)
  line L2 (159.7, 244) -> (60.3, 244)
  line L3 (60.3, 244) -> (60.3, 240)
  dimension "d1468" = 240
  dimension "d1469" = 99.4
  dimension "d1470" = 4
  constraint horizontal L0
  constraint vertical L1
  constraint horizontal L2
  constraint vertical L3
  measures "d1468" vertical distance of origin L0.start
  measures "d1469" horizontal distance of L0.start L0.end
  measures "d1470" vertical distance of L0.end L1.end
extrude "Drain slot 7''''" cut sketch "草图8 (10)" along normal blind 4 bodies 26 in component "LS_RemovableGrate"
ref_plane "工作平面9" through (0, 0, 36) normal (0, 0, 1) x (1, 0, 0) in component "LS_RemovableGrate"
sketch "草图9 (10)" plane through (0, 0, 36) normal (0, 0, 1) x (1, 0, 0) in component "LS_RemovableGrate"
  line L0 (60.3, 230) -> (159.7, 230)
  line L1 (159.7, 230) -> (159.7, 234)
  line L2 (159.7, 234) -> (60.3, 234)
  line L3 (60.3, 234) -> (60.3, 230)
  dimension "d1476" = 230
  dimension "d1477" = 99.4
  dimension "d1478" = 4
  constraint horizontal L0
  constraint vertical L1
  constraint horizontal L2
  constraint vertical L3
  measures "d1476" vertical distance of origin L0.start
  measures "d1477" horizontal distance of L0.start L0.end
  measures "d1478" vertical distance of L0.end L1.end
extrude "Drain slot 8''''" cut sketch "草图9 (10)" along normal blind 4 bodies 26 in component "LS_RemovableGrate"
ref_plane "工作平面10" through (0, 0, 36) normal (0, 0, 1) x (1, 0, 0) in component "LS_RemovableGrate"
sketch "草图10 (10)" plane through (0, 0, 36) normal (0, 0, 1) x (1, 0, 0) in component "LS_RemovableGrate"
  line L0 (60.3, 220) -> (159.7, 220)
  line L1 (159.7, 220) -> (159.7, 224)
  line L2 (159.7, 224) -> (60.3, 224)
  line L3 (60.3, 224) -> (60.3, 220)
  dimension "d1484" = 220
  dimension "d1485" = 99.4
  dimension "d1486" = 4
  constraint horizontal L0
  constraint vertical L1
  constraint horizontal L2
  constraint vertical L3
  measures "d1484" vertical distance of origin L0.start
  measures "d1485" horizontal distance of L0.start L0.end
  measures "d1486" vertical distance of L0.end L1.end
extrude "Drain slot 9''''" cut sketch "草图10 (10)" along normal blind 4 bodies 26 in component "LS_RemovableGrate"
ref_plane "工作平面11" through (0, 0, 36) normal (0, 0, 1) x (1, 0, 0) in component "LS_RemovableGrate"